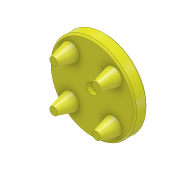
# Autodesk Inventor part: ground_support_2
Saved by Autodesk Inventor 2018 (Build 220112000, 112)
## iProperties
Created: 2019-12-28
Part Number: ground_support_2
Material: Generic
Document SubType Name: Modeling
Designer: nnico
Density: 1 g/cm^3
Appearance: Yellow
Author: nnico
## iProperties of the stored document base2_3DPrint.ipt
Created: 2020-03-25
Part Number: base2_3DPrint
Material: Generic
Document SubType Name: Modeling
Designer: nnico
Density: 1 g/cm^3
Appearance: Default
Author: nnico
Autodesk Inventor part; units mm, degrees
ref_plane "YZ Plane" through (0, 0, 0) normal (1, 0, 0) x (0, 1, 0)
ref_plane "XZ Plane" through (0, 0, 0) normal (0, 1, 0) x (-1, 0, 0)
ref_plane "XY Plane" through (0, 0, 0) normal (0, 0, 1) x (1, 0, 0)
sketch "Sketch1" plane through (0, 0, 0) normal (0, 1, 0) x (-1, 0, 0)
  circle A0 centre (0, 0) radius 50
  circle A1 centre (0, 0) radius 6.25
  dimension "d0" = 100
  dimension "d1" = 12.5
  constraints: 2 centre point, 2 coincident
  measures "d0" diameter of A0
  measures "d1" diameter of A1
extrude "Extrusion1" add sketch "Sketch1" along normal blind 5
sketch "Sketch2" plane through (0, 5, 0) normal (0, 1, 0) x (1, 0, 0)
  line L0 (9.75, 0) -> (4.875, -8.4437)
  line L1 (4.875, -8.4437) -> (-4.875, -8.4437)
  line L2 (-4.875, -8.4437) -> (-9.75, 0)
  line L3 (-9.75, 0) -> (-4.875, 8.4437)
  line L4 (-4.875, 8.4437) -> (4.875, 8.4437)
  line L5 (4.875, 8.4437) -> (9.75, 0)
  line L6 (0, 0) -> (0, 50) construction
  circle A0 centre (0, 0) radius 50 construction
  line L7 (0, 0) -> (-50, 0) construction
  circle A1 centre (0, 0) radius 15
  dimension "d4" = 19.5
  dimension "d5" = 30
  constraints: 16 end point, 2 coincident, 2 perpendicular, 2 point on circle, 1 centre point, 1 vertical, 13 other
  measures "d4" distance of L0.start L2.end
  measures "d5" diameter of A1
extrude "Extrusion2" add sketch "Sketch2" along normal blind 10
sketch "Sketch3" plane through (0, 5, 0) normal (0, 1, 0) x (1, 0, 0)
  circle A0 centre (0, 0) radius 50
  circle A1 centre (0, 0) radius 47.5
  dimension "d8" = 95
  constraints: 2 centre point, 2 coincident
  measures "d8" diameter of A1
extrude "Extrusion3" add sketch "Sketch3" along normal blind 5
sketch "Sketch4" plane through (0, 10, 0) normal (0, 1, 0) x (1, 0, 0)
  circle A0 centre (0, 0) radius 15
  circle A1 centre (0, 0) radius 50
  constraints: 2 centre point, 2 coincident
extrude "Extrusion4" add sketch "Sketch4" along normal blind 5
sketch "Sketch5" plane through (0, 0, 0) normal (0, -1, 0) x (1, 0, 0)
  circle A0 centre (0, 0) radius 6.25 construction
  line L0 (0, 0) -> (0, -50) construction
  circle A1 centre (0, 0) radius 50 construction
  line L1 (0, 0) -> (50, 0) construction
  circle A2 centre (25, -25) radius 10
  circle A3 centre (-25, -25) radius 10
  circle A4 centre (25, 25) radius 10
  circle A5 centre (-25, 25) radius 10
  dimension "d13" = 20
  dimension "d14" = 25
  dimension "d15" = 25
  constraints: 4 centre point, 4 end point, 3 symmetric about line, 2 point on circle, 1 perpendicular, 1 vertical, 3 other
  measures "d13" diameter of A2
  measures "d14" distance from line of L0 A2.centre
  measures "d15" distance from line of L1 A2.centre
extrude "Extrusion5" add sketch "Sketch5" along normal blind 20
draft "FaceDraft1" angle 15 pull direction (0, -1, 0) faces at (34.8705, -13.3333, -26.6041) fixed edges at (15, 0, -25)
draft "FaceDraft3" angle 15 pull direction (0, -1, 0) faces at (-15.1295, -13.3333, -26.6041) fixed edges at (-35, 0, -25)
draft "FaceDraft4" angle 15 pull direction (0, -1, 0) faces at (34.8705, -13.3333, 23.3959) fixed edges at (15, 0, 25)
draft "FaceDraft5" angle 15 pull direction (0, -1, 0) faces at (-15.1295, -13.3333, 23.3959) fixed edges at (-35, 0, 25)
chamfer "Chamfer1" distance 2 angle 45 1 edges at (-50, 15, 0)
chamfer "Chamfer2" distance 2 angle 45 1 edges at (50, 0, 0)
body "Solid1"
